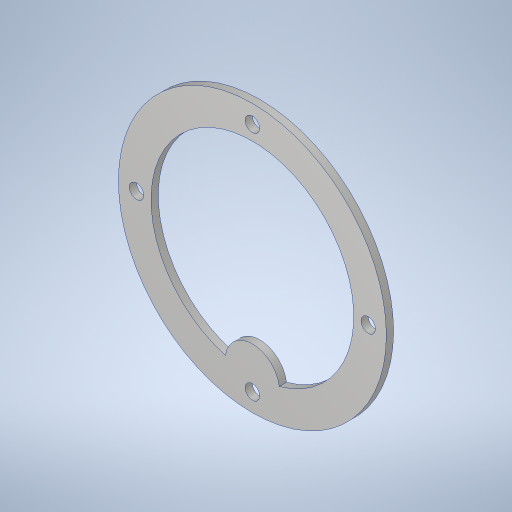
# Autodesk Inventor part: Gasket
Saved by Autodesk Inventor 2023.4 (Build 274418000, 418)
## iProperties
Created: 2025-02-28
Part Number: Gasket
Material: Aluminum 6061
Document SubType Name: Modeling
Designer: jmcintyr
Density: 2.7 g/cm^3
Appearance: Aluminum - Flat
Author: jmcintyr
Autodesk Inventor part; units mm, degrees
ref_plane "YZ Plane" through (0, 0, 0) normal (1, 0, 0) x (0, 1, 0)
ref_plane "XZ Plane" through (0, 0, 0) normal (0, 1, 0) x (-1, 0, 0)
ref_plane "XY Plane" through (0, 0, 0) normal (0, 0, 1) x (1, 0, 0)
sketch "Sketch1" plane through (0, 0, 0) normal (0, 0, 1) x (1, 0, 0)
  arc A0 (9.4392, -34.2843) -> (-9.4392, -34.2843) centre (0, 0) ccw
  circle A1 centre (0, 0) radius 46.99
  arc A2 (9.4392, -34.2843) -> (-9.4392, -34.2843) centre (0, -35.56) ccw
  circle A3 centre (0, 40.64) radius 2.5527
  circle A4 centre (-40.64, 0) radius 2.5527
  circle A5 centre (0, -40.64) radius 2.5527
  circle A6 centre (40.64, 0) radius 2.5527
  point P0 (0, 46.99)
  dimension "d1" = 93.98
  dimension "d0" = 71.12
  dimension "d2" = 19.05
  dimension "d8" = 360
  dimension "d12" = 5.1054
  dimension "d13" = 6.35
  constraints: 6 centre point, 5 point on circle, 4 vertical alignment, 2 coincident, 11 other
  measures "d0" diameter of A0
  measures "d2" diameter of A2
  measures "d12" diameter of A3
  measures "d13" distance of A3.centre point (0, 46.99)
extrude "Extrusion1" add sketch "Sketch1" along normal blind 2.54
body "Solid1"
